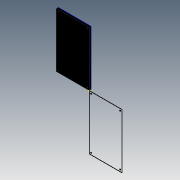
# Autodesk Inventor part: sideplate_top
Saved by Autodesk Inventor 2015 (Build 190159000, 159)
## iProperties
Created: 2014-08-31
Part Number: sideplate_top
Material: Generic
Document SubType Name: Modeling
Designer: shohei
Density: 1 g/cm^3
Appearance: Default
Mass: 540 g
Surface Area: 1176 cm^2
Volume: 540 cm^3
Author: shohei
Autodesk Inventor part; units mm, degrees
ref_plane "YZ Plane" through (0, 0, 0) normal (1, 0, 0) x (0, 1, 0)
ref_plane "XZ Plane" through (0, 0, 0) normal (0, 1, 0) x (-1, 0, 0)
ref_plane "XY Plane" through (0, 0, 0) normal (0, 0, 1) x (1, 0, 0)
sketch "Block1" plane through (0, 0, 0) normal (0, 0, 1) x (1, 0, 0)
  line L0 (-180.22, 0.22) -> (0.22, 0.22)
  line L1 (0.22, 0.22) -> (0.22, -300.22)
  line L2 (0.22, -300.22) -> (-180.22, -300.22)
  line L3 (-180.22, -300.22) -> (-180.22, 0.22)
  circle A0 centre (-170, -10) radius 2.72
  circle A1 centre (-10, -10) radius 2.72
  circle A2 centre (-170, -290) radius 2.72
  circle A3 centre (-10, -290) radius 2.72
  point P0 (-90, -150)
sketch "Sketch1" plane through (0, 0, 0) normal (0, 1, 0) x (-1, 0, 0)
  line L0 (0, 0) -> (180, 0)
  line L1 (180, 0) -> (180, 300)
  line L2 (180, 300) -> (0, 300)
  line L3 (0, 300) -> (0, 0)
  circle A0 centre (170, 10) radius 2.5
  line L4 (90, -51.0064) -> (90, 353.269)
  line L5 (216.4039, 150) -> (-14.4683, 150)
  circle A1 centre (10, 10) radius 2.5
  circle A2 centre (170, 290) radius 2.5
  circle A3 centre (10, 290) radius 2.5
  dimension "d0" = 180
  dimension "d1" = 300
  dimension "d4" = 5
  dimension "d5" = 10
  dimension "d6" = 10
  dimension "d7" = 90
  dimension "d8" = 150
  constraints: 12 end point, 4 centre point, 3 symmetric about line, 2 horizontal, 2 parallel, 1 perpendicular, 1 vertical, 3 other
  measures "d0" distance of L1.end L2.end
  measures "d1" distance of L0.end L1.end
  measures "d4" diameter of A0
  measures "d5" distance from line of L1 A0.centre
  measures "d6" distance from line of L0 A0.centre
  measures "d7" distance between parallel lines of L1 L4
  measures "d8" distance between parallel lines of L0 L5
extrude "Extrusion2" add sketch "Sketch1" along normal blind 10
sketch "Sketch2" plane through (0, 10, 0) normal (0, 1, 0) x (1, 0, 0)
  circle A0 centre (-10, -290) radius 2.5 projected
  circle A1 centre (-170, -290) radius 2.5 projected
  circle A2 centre (-10, -10) radius 2.5 projected
  circle A3 centre (-170, -10) radius 2.5 projected
  line L0 (0, 0) -> (-180, 0) projected
  line L1 (-180, 0) -> (-180, -300) projected
  line L2 (-180, -300) -> (0, -300) projected
  line L3 (0, -300) -> (0, 0) projected
  constraints: 3 perpendicular, 4 other
sketch "DXF" plane through (0, 0, 0) normal (0, 1, 0) x (-1, 0, 0)
  point P0 (0, 0)
body "Solid2"
